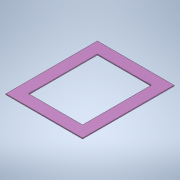
# Autodesk Inventor part: Fomi
Saved by Autodesk Inventor 2022.6 (Build 266554000, 554)
## iProperties
Created: 2025-01-16
Part Number: Fomi
Material: Genérico
Document SubType Name: Modeling
Designer: johan
Density: 1 g/cm^3
Appearance: Valor por defecto
Author: johan
Autodesk Inventor part; units mm, degrees
ref_plane "YZ Plane" through (0, 0, 0) normal (1, 0, 0) x (0, 1, 0)
ref_plane "XZ Plane" through (0, 0, 0) normal (0, 1, 0) x (-1, 0, 0)
ref_plane "XY Plane" through (0, 0, 0) normal (0, 0, 1) x (1, 0, 0)
sketch "Boceto1" plane through (0, 0, 0) normal (0, 1, 0) x (-1, 0, 0)
  line L0 (0, 0) -> (243, 0)
  line L1 (243, 0) -> (243, -290)
  line L2 (243, -290) -> (0, -290)
  line L3 (0, -290) -> (0, 0)
  line L4 (207, -254) -> (207, -36)
  line L5 (207, -36) -> (36, -36)
  line L6 (36, -36) -> (36, -254)
  line L7 (36, -254) -> (207, -254)
  dimension "d0" = 243
  dimension "d1" = 290
  dimension "d2" = 36
  constraints: 16 end point, 4 parallel, 2 perpendicular, 1 horizontal, 3 other
  measures "d0" distance of L1.end L2.end
  measures "d1" distance of L0.end L1.end
  measures "d2" distance between parallel lines of L1 L4
extrude "Extrusión1" add sketch "Boceto1" along normal blind 3
